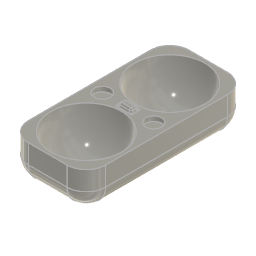
Silicon ear plugs case v8 (Autodesk Fusion 360 design; units mm, degrees)
Autodesk Fusion 360 part; units mm, degrees
note: some values were not read from the file. Chosen so that the rebuilt part matches the saved one: which pieces of a blend or face edit are solid.
sketch "Sketch1" plane through (0, 0, 0) normal (0, 0, 1) x (1, 0, 0)
  line L0 (12, -25) -> (-12, -25)
  line L1 (-12, -25) -> (-12, 25)
  line L2 (-12, 25) -> (12, 25)
  line L3 (12, 25) -> (12, -25)
  line L4 (12, -25) -> (-12, 25) construction
  line L5 (-12, -25) -> (12, 25) construction
  dimension "d1" = 24
  dimension "d2" = 50
  constraint horizontal L0
  constraint perpendicular L0 L1
  constraint parallel L0 L2
  constraint parallel L1 L3
  constraint coincident L4 origin
  constraint coincident L5 origin
  measures "d1" distance of L1.end L2.end
  measures "d2" distance of L0.end L1.end
extrude "Extrude1" add sketch "Sketch1" along normal blind 12 makes body 1
sketch "Sketch2" plane through (0, 0, 12) normal (0, 0, 1) x (-1, 0, 0)
  line L0 (-12, -25) -> (12, -25)
  line L1 (12, -25) -> (12, 25)
  line L2 (12, 25) -> (-12, 25)
  line L3 (-12, 25) -> (-12, -25)
sketch "Sketch3" plane through (0, 0, 12) normal (0, 0, 1) x (-1, 0, 0)
  point P0 (0, -13)
  point P1 (0, 13)
sketch "Sketch4" plane through (0, 0, 12) normal (0, 0, 1) x (-1, 0, 0)
sphere "SpherePrimitive1" cut diameter 22 placed x (-1, 0, 0) y (0, -1, 0) z (0, 0, 1) at (0, -13, 12) bodies 1
sphere "SpherePrimitive2" cut diameter 22 placed x (-1, 0, 0) y (0, -1, 0) z (0, 0, 1) at (0, 13, 12) bodies 1
sketch "Sketch6" plane through (0, 0, 12) normal (0, 0, 1) x (-1, 0, 0)
  circle A0 centre (-8, 0) radius 2.5
  dimension "d7" = 5
  measures "d7" diameter of A0
sketch "Sketch7" plane through (0, 0, 12) normal (0, 0, 1) x (1, 0, 0)
  circle A0 centre (-8, 0) radius 2.5
  dimension "d8" = 5
  measures "d8" diameter of A0
extrude "Extrude2" cut sketch "Sketch7" against normal blind 1.5 bodies 1
extrude "Extrude3" cut sketch "Sketch6" against normal blind 1.5 bodies 1
sketch "Sketch8" plane through (0, 0, 12) normal (0, 0, 1) x (-1, 0, 0)
  line L0 (-2, 1) -> (2, 1)
  line L1 (2, 1) -> (2, -1)
  line L2 (2, -1) -> (-2, -1)
  line L3 (-2, -1) -> (-2, 1)
  dimension "d13" = 4
  constraint horizontal L0
  constraint vertical L1
  constraint horizontal L2
  constraint vertical L3
  measures "d13" distance of L0.start L0.end
extrude "Extrude4" add sketch "Sketch8" along normal blind 1 bodies 1
fillet "Fillet1" radius 6 1 edges at (12, -25, 6) on bodies 1
fillet "Fillet2" radius 6 1 edges at (-12, -25, 6) on bodies 1
fillet "Fillet3" radius 6 1 edges at (12, 25, 6) on bodies 1
fillet "Fillet4" radius 6 1 edges at (-12, 25, 6) on bodies 1
fillet "Fillet5" radius 6 8 edges at (-12, 0, 0) (-10.2426, -23.2426, 0) (0, -25, 0) (10.2426, -23.2426, 0) (12, 0, 0) (10.2426, 23.2426, 0) (0, 25, 0) (-10.2426, 23.2426, 0) on bodies 1
fillet "Fillet6" radius 0.5 1 edges at (0, 1, 13) on bodies 1
fillet "Fillet7" radius 0.5 1 edges at (0, -1, 13) on bodies 1
fillet "Fillet8" radius 0.5 5 edges at (-2, 1, 12.25) (-2, 0.8536, 12.8536) (-2, 0, 13) (-2, -0.8536, 12.8536) (-2, -1, 12.25) on bodies 1
fillet "Fillet9" radius 0.5 5 edges at (2, -1, 12.25) (2, -0.8536, 12.8536) (2, 0, 13) (2, 0.8536, 12.8536) (2, 1, 12.25) on bodies 1
fillet "Fillet10" radius 0.5 8 edges at (-1.8536, -0.8536, 12) (-2, 0, 12) (-1.8536, 0.8536, 12) (0, 1, 12) (1.8536, 0.8536, 12) (2, 0, 12) (1.8536, -0.8536, 12) (0, -1, 12) on bodies 1
copy_body "CopyPasteBodies1" bodies 1 makes body 2
move_face "OffsetFaces1" offset -1 1 faces at (0.5, -0.1667, 13) on bodies 2
sketch "Sketch9" plane through (0, 0, 12) normal (0, 0, 1) x (-1, 0, 0)
extrude "Extrude5" cut sketch "Sketch8" against normal blind 1 bodies 2
fillet "Fillet11" radius 0.5 1 edges at (2, 0, 12) on bodies 2
fillet "Fillet12" radius 0.5 1 edges at (0.25, -1, 12) on bodies 2
fillet "Fillet13" radius 0.5 1 edges at (-2, -0.25, 12) on bodies 2
fillet "Fillet14" radius 0.5 1 edges at (0, 1, 12) on bodies 2
fillet "Fillet15" radius 0.5 1 edges at (0, 1, 11) on bodies 2
fillet "Fillet16" radius 0.5 3 edges at (2.1464, 1.1464, 11.8536) (2, 0.8536, 11.1464) (2, -0.25, 11) on bodies 2
fillet "Fillet17" radius 0.5 3 edges at (2.1464, -1.1464, 11.8536) (1.8536, -1, 11.1464) (-0.25, -1, 11) on bodies 2
fillet "Fillet18" radius 0.5 5 edges at (-2.1464, -1.1464, 11.8536) (-2, -0.8536, 11.1464) (-2, 0, 11) (-2, 0.8536, 11.1464) (-2.1464, 1.1464, 11.8536) on bodies 2
move_body "Move1" bodies 2 to x (1, 0, 0) y (0, 1, 0) z (0, 0, 1) at (39, 0, 0)
move_body "Align1" bodies 2 to x (1, 0, 0) y (0, 1, 0) z (0, 0, 1) at (-39, 0, 0)
